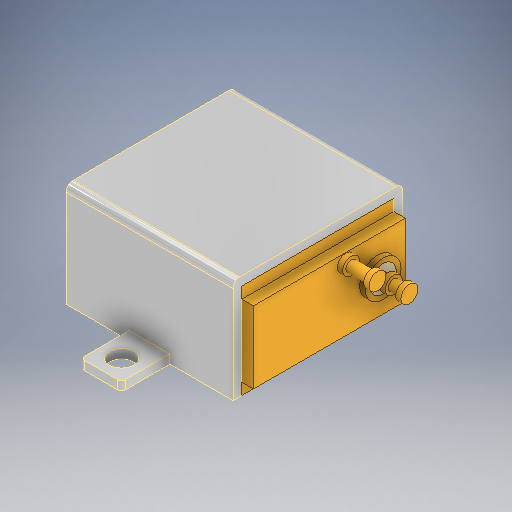
# Autodesk Inventor part: Mini-Circuits_Case_GC957
Saved by Autodesk Inventor 2025.2 (Build 292293000, 293)
## iProperties
Created: 2024-11-19
Part Number: Mini-Circuits_Case_GC957
Material: Generic
Document SubType Name: Modeling
Designer: Paul Linke
Density: 1 g/cm^3
Appearance: Gold
Author: Paul Linke
Autodesk Inventor part; units mm, degrees
ref_plane "YZ Plane" through (0, 0, 0) normal (1, 0, 0) x (0, 1, 0)
ref_plane "XZ Plane" through (0, 0, 0) normal (0, 1, 0) x (-1, 0, 0)
ref_plane "XY Plane" through (0, 0, 0) normal (0, 0, 1) x (1, 0, 0)
sketch "sketch_main_body" plane through (0, 0, 0) normal (0, 1, 0) x (-1, 0, 0)
  line L0 (9.4, -8.55) -> (-9.4, -8.55)
  line L1 (-9.4, -8.55) -> (-9.4, 8.55)
  line L2 (-9.4, 8.55) -> (9.4, 8.55)
  line L3 (9.4, 8.55) -> (9.4, -8.55)
  line L4 (9.4, -8.55) -> (-9.4, 8.55) construction
  line L5 (-9.4, -8.55) -> (9.4, 8.55) construction
  point P0 (0, 0)
  dimension "d0" = 18.8
  dimension "d1" = 17.1
  constraints: 12 end point, 2 midpoint, 2 parallel, 1 horizontal, 1 perpendicular
  measures "d0" distance between parallel lines of L1 L3
  measures "d1" distance between parallel lines of L2 L0
extrude "main_body" add sketch "sketch_main_body" along normal blind 10.68
sketch "sketch_aluminium_shield" plane through (-9.4, 0, -8.55) normal (-1, 0, 0) x (0, 0, 1)
  line L0 (0, 0) -> (0, 10.68) projected
  line L1 (0, 0) -> (-1, 0)
  line L2 (-1, 0) -> (-1, 10.93)
  line L3 (-0.25, 11.68) -> (0.0237, 11.68)
  line L4 (0, 10.68) -> (0, 0)
  line L5 (0.0237, 11.68) -> (17.35, 11.68)
  line L6 (18.1, 10.93) -> (18.1, 10.5311)
  line L7 (17.1, 10.68) -> (0, 10.68)
  line L8 (17.1, 0) -> (17.1, 10.68) projected
  line L9 (17.1, 10.5311) -> (17.1, 0)
  line L10 (17.1, 0) -> (18.1, 0)
  line L11 (18.1, 0) -> (18.1, 10.68)
  arc A0 (-0.25, 11.68) -> (-1, 10.93) centre (-0.25, 10.93) ccw
  arc A1 (18.1, 10.93) -> (17.35, 11.68) centre (17.35, 10.93) ccw
  point P0 (8.55, 0)
  dimension "d5" = 1
  dimension "d6" = 1
  dimension "d7" = 1
  dimension "d8" = 0.75
  constraints: 20 end point, 4 parallel, 4 point on circle, 4 tangent, 3 horizontal, 3 point on line, 2 centre point, 2 perpendicular, 1 equal radius
  measures "d5" distance between parallel lines of L0 L2
  measures "d6" distance between parallel lines of L5 L7
  measures "d7" distance between parallel lines of L11 L8
  measures "d8" radius of A0
extrude "aluminium_shield" add sketch "sketch_aluminium_shield" against normal blind 18.8 separate body
sketch "sketch_mount" plane through (0, 0, 0) normal (0, -1, 0) x (1, 0, 0)
  line L0 (-9.4, 9.55) -> (9.4, 9.55) projected
  line L1 (-2.285, 9.55) -> (2.285, 9.55)
  line L2 (2.285, 9.55) -> (2.285, 14.6)
  line L3 (1.885, 15) -> (-1.885, 15)
  line L4 (-2.285, 14.6) -> (-2.285, 9.55)
  circle A0 centre (0, 12.7) radius 1.345
  arc A1 (-1.885, 15) -> (-2.285, 14.6) centre (-1.885, 14.6) ccw
  arc A2 (2.285, 14.6) -> (1.885, 15) centre (1.885, 14.6) ccw
  line L5 (-12.1941, 0) -> (12.1129, 0) construction
  line L6 (-9.4, -9.55) -> (9.4, -9.55)
  line L7 (2.285, -9.55) -> (2.285, -14.6)
  line L8 (1.885, -15) -> (-1.885, -15)
  line L9 (-2.285, -14.6) -> (-2.285, -9.55)
  circle A3 centre (0, -12.7) radius 1.345
  arc A4 (-2.285, -14.6) -> (-1.885, -15) centre (-1.885, -14.6) ccw
  arc A5 (1.885, -15) -> (2.285, -14.6) centre (1.885, -14.6) ccw
  point P0 (0, 0)
  point P1 (0, 9.55)
  point P2 (2.285, 9.55)
  dimension "d11" = 5.45
  dimension "d12" = 4.57
  dimension "d14" = 7.115
  dimension "d15" = 0.4
  dimension "d16" = 2.69
  dimension "d17" = 3.15
  constraints: 18 end point, 11 symmetric about line, 8 point on circle, 6 centre point, 4 tangent, 2 horizontal, 2 parallel, 2 point on line, 1 equal radius, 1 midpoint, 1 perpendicular, 3 other
  measures "d11" distance between parallel lines of L0 L3
  measures "d12" distance between parallel lines of L2 L4
  measures "d14" distance from line of L0.end L2
  measures "d15" radius of A1
  measures "d16" diameter of A0
  measures "d17" distance of point (0, 9.55) A0.centre
extrude "mount" add sketch "sketch_mount" against normal blind 1 bodies 2
sketch "sketch_bulge" plane through (9.4, 0, 8.55) normal (1, 0, 0) x (0, 0, -1)
  line L0 (0, 0) -> (0, 10.68) projected
  line L1 (17.1, 0) -> (17.1, 10.68) projected
  line L2 (0, 9.39) -> (17.1, 9.39)
  line L3 (17.1, 9.39) -> (17.1, 1.29)
  line L4 (17.1, 1.29) -> (0, 1.29)
  line L5 (0, 1.29) -> (0, 9.39)
  line L6 (0, 10.68) -> (17.1, 10.68) projected
  point P0 (8.55, 0)
  point P1 (0, 1.29)
  dimension "d20" = 8.1
  dimension "d21" = 1.29
  constraints: 8 end point, 2 parallel, 2 point on line, 1 horizontal, 1 perpendicular
  measures "d20" distance between parallel lines of L4 L2
  measures "d21" distance between parallel lines of L6 L2
extrude "bulge" add sketch "sketch_bulge" along normal blind 1.3 contours L0 L2 L1 L4 bodies 1
sketch "sketch_power_ports" plane through (10.7, 0, 8.55) normal (1, 0, 0) x (0, 0, -1)
  circle A0 centre (13.99, 5.33) radius 0.95
  circle A1 centre (13.99, 5.33) radius 0.6
  line L0 (0, 0) -> (17.1, 0) projected
  circle A2 centre (13.99, 5.33) radius 2.02
  line L1 (-1, 10.93) -> (-1, 0) projected
  circle A3 centre (10.4, 8.38) radius 0.95
  circle A4 centre (10.4, 8.38) radius 0.6
  circle A5 centre (13.99, 5.33) radius 1.48
  point P0 (8.55, 0)
  dimension "d24" = 1.2
  dimension "d25" = 1.9
  dimension "d26" = 5.33
  dimension "d27" = 4.04
  dimension "d28" = 14.99
  dimension "d29" = 1.2
  dimension "d30" = 1.9
  dimension "d31" = 8.38
  dimension "d32" = 11.4
  dimension "d45" = 2.96
  constraints: 6 centre point, 5 coincident
  measures "d24" diameter of A1
  measures "d25" diameter of A0
  measures "d26" distance from line of A0.centre L0
  measures "d27" diameter of A2
  measures "d28" distance from line of A0.centre L1
  measures "d29" diameter of A4
  measures "d30" diameter of A3
  measures "d31" distance from line of A3.centre L0
  measures "d32" distance from line of A3.centre L1
  measures "d45" diameter of A5
extrude "Extrusion5" add sketch "sketch_power_ports" along normal blind 3.56 contours A4 bodies 1
extrude "Extrusion6" add sketch "sketch_power_ports" along normal blind 0.6 from surface at 0 contours A3 | A4 bodies 1
extrude "Extrusion7" add sketch "sketch_power_ports" against normal blind 0.6 from surface at 3.56 contours A3 | A4 bodies 1
extrude "Extrusion9" add sketch "sketch_power_ports" along normal blind 3.56 contours A1 bodies 1
extrude "Extrusion11" add sketch "sketch_power_ports" along normal blind 0.6 separate body contours A0 | A5
extrude "Extrusion12" add sketch "sketch_power_ports" along normal blind 0.6 contours A2 bodies 1
extrude "Extrusion13" add sketch "sketch_power_ports" against normal blind 0.6 from surface at 3.56 contours A0 bodies 1
extrude "Extrusion14" add sketch "sketch_power_ports" along normal blind 1.2 from surface at 0.6 contours A0 bodies 1
extrude "Extrusion15" cut sketch "sketch_power_ports" along normal blind 1.2 contours A0 bodies 1
body "Solid1"
body "Solid2"
body "Solid3"
